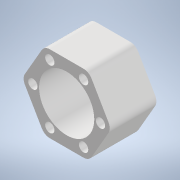
# Autodesk Inventor part: EndBearingMountSpacer
Saved by Autodesk Inventor 2020 (Build 240168000, 168)
## iProperties
Created: 2020-01-23
Part Number: EndBearingMountSpacer
Material: Generic
Document SubType Name: Modeling
Designer: srini
Density: 1 g/cm^3
Appearance: Default
Author: srini
Autodesk Inventor part; units mm, degrees
ref_plane "YZ Plane" through (0, 0, 0) normal (1, 0, 0) x (0, 1, 0)
ref_plane "XZ Plane" through (0, 0, 0) normal (0, 1, 0) x (-1, 0, 0)
ref_plane "XY Plane" through (0, 0, 0) normal (0, 0, 1) x (1, 0, 0)
sketch "Sketch1" plane through (0, 0, 0) normal (0, 0, 1) x (1, 0, 0)
  line L0 (-25.4, -50.5029) -> (-25.4, -85.7859) projected
  line L1 (-25.4, -85.7859) -> (-23.8734, -87.3125) projected
  line L2 (-23.8734, -87.3125) -> (-1.5266, -87.3125) projected
  line L3 (-1.5266, -87.3125) -> (0, -85.7859) projected
  line L4 (0, -85.7859) -> (0, -50.5029) projected
  arc A0 (0.5036, -48.0245) -> (0, -50.5029) centre (6.35, -50.5029) ccw construction
  line L5 (0.5036, -48.0245) -> (11.5821, -21.8911) construction
  line L6 (11.5821, -21.8911) -> (11.5821, -19.7321) construction
  line L7 (11.5821, -19.7321) -> (0.8961, -1.5266) construction
  line L8 (0.8961, -1.5266) -> (-0.6306, 0) construction
  line L9 (-0.6306, 0) -> (-24.7694, 0) construction
  line L10 (-26.2961, -1.5266) -> (-24.7694, 0) construction
  line L11 (-26.2961, -1.5266) -> (-36.9821, -19.7321) construction
  line L12 (-36.9821, -19.7321) -> (-36.9821, -21.8911) construction
  line L13 (-36.9821, -21.8911) -> (-25.9036, -48.0245) construction
  arc A1 (-25.4, -50.5029) -> (-25.9036, -48.0245) centre (-31.75, -50.5029) ccw construction
  circle A2 centre (-3.4925, -4.6896) radius 2.0701 construction
  circle A3 centre (5.715, -20.6375) radius 2.0701 construction
  circle A4 centre (-12.7, -80.9625) radius 2.0701 projected
  circle A5 centre (-12.7, -55.5625) radius 2.0701 construction
  circle A6 centre (-12.7, -20.6375) radius 14.2875 construction
  circle A7 centre (-12.7, -42.8625) radius 2.0701 construction
  circle A8 centre (-12.7, -68.2625) radius 2.0701 construction
  circle A9 centre (-31.115, -20.6375) radius 2.0701 construction
  circle A10 centre (-21.9075, -4.6896) radius 2.0701 construction
  line L14 (5.715, -20.6375) -> (-31.115, -20.6375) construction
  circle A11 centre (-3.4925, -4.6896) radius 2.54
  circle A12 centre (-21.9075, -4.6896) radius 2.54
  circle A13 centre (-31.115, -20.6375) radius 2.54
  circle A14 centre (5.715, -20.6375) radius 2.54
  circle A15 centre (-3.4925, -36.5854) radius 2.54
  circle A16 centre (-21.9075, -36.5854) radius 2.54
  line L15 (11.5231, -20.6375) -> (-0.5884, -41.6154)
  line L16 (-0.5884, -41.6154) -> (-24.8116, -41.6154)
  line L17 (-24.8116, -41.6154) -> (-36.9231, -20.6375)
  line L18 (-36.9231, -20.6375) -> (-24.8116, 0.3404)
  line L19 (-24.8116, 0.3404) -> (-0.5884, 0.3404)
  line L20 (-0.5884, 0.3404) -> (11.5231, -20.6375)
  circle A17 centre (-12.7, -20.6375) radius 15.015
  circle A18 centre (5.715, -20.6375) radius 3.4 construction
  circle A19 centre (5.715, -20.6375) radius 5.03
  point P0 (0, 0)
  dimension "d0" = 5.08
  dimension "d6" = 36.83
  dimension "d7" = 6.8
  dimension "d8" = 10.06
  constraints: 14 end point, 9 centre point, 8 coincident, 3 equal radius, 2 horizontal, 2 symmetric about line, 2 tangent, 15 other
  measures "d0" diameter of A13
  measures "d6" distance of L14.start L14.end
  measures "d7" diameter of A18
  measures "d8" diameter of A19
extrude "Extrusion1" add sketch "Sketch1" along normal blind 25.4 contours L15 A19 L20 | L15 L16 L17 L18 L19 L20 A19 A17 | A19 A17 picked at (3.083, -23.4499)
fillet "Fillet1" radius 5.03 6 edges at (-0.5884, 0.3404, 12.7) (-24.8116, 0.3404, 12.7) (-36.9231, -20.6375, 12.7) (-24.8116, -41.6154, 12.7) (-0.5884, -41.6154, 12.7) (11.5231, -20.6375, 12.7)
equation "\"d5\" = 0.5 * d8"
body "Solid1"
